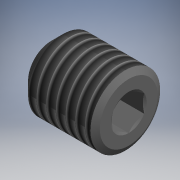
# Autodesk Inventor part: DIN-913 - M18x20
Saved by Autodesk Inventor 2017.3 (Build 213256000, 256)
## iProperties
Part Number: DIN-913 - M18x20
Material: Generic
Catalog Web Link: www.cadenas.de
Description: DIN-913-Gewindestift
Vendor: FESTO
Document SubType Name: Modeling
Designer: partserver
Manufacturer: FESTO
Mass: 4.27109 g
Surface Area: 17.6345 cm^2
Volume: 4.27109 cm^3
Density: 1 g/cm^3
Appearance: PSOLRGB-128-128-128
Category: PARTsolutions
Company: FESTO
Title: DIN-913 - M18x20
Author: Cadenas PARTsolutions
Comments: Gewindestift
PSOL_IDENT_0: {$CADENAS_DATA\23d-libs\festo\zyl_zubeh\din_913\din_913.prj},177 {VTYP=3D},{NB=DIN-913 - M18x20},{LI
PSOL_IDENT_1: NA=DIN-913 - M18x20},{NN=DIN-913},{DATE=22.07.2016 11:33:17},{GEOMDATE=22.07.2016 11:33:13},{VERSION=
PSOL_IDENT_2: v3},{LINEID=1120},{WBVAR=},{WBNUMERIC=}  {NB=DIN-913 - M18x20},{LINA=DIN-913 - M18x20},{KT=X},{IDNR=
PSOL_IDENT_3: },{NENN=M18x20},{D=18.000},{D3=14.933},{P=2.500},{L=20.000},{DP=12.000},{S=8.000},{T=10.000}
NB: DIN-913 - M18x20
NN: DIN-913
NT: Gewindestift
NBSYN: DIN-913 - $NENN.
LINA: DIN-913 - M18x20
CATALOG: Festo
ROWDESC: M18x20
D: 18
D3: 14.933
P: 2.5
L: 20
DP: 12
S: 8
T: 10
SUPPLIER: FESTO
ARTICLENO: DIN-913 - M18x20
BOMINFO: DIN-913 - M18x20
CREATOR: CADENAS GmbH
Autodesk Inventor part; units mm, degrees
sketch "Sketch_1" plane through (0, 0, 0) normal (0, 0, 1) x (1, 0, 0)
  line L0 (2.6667, 0) -> (20, 0)
  line L1 (20, 0) -> (20, -6)
  line L2 (20, -6) -> (17, -9)
  line L3 (17, -9) -> (0.8854, -9)
  line L4 (0.8854, -9) -> (0, -7.4665)
  line L5 (0, -7.4665) -> (0, -4.6188)
  line L6 (0, -4.6188) -> (2.6667, 0)
  line L7 (2.6667, 0) -> (20, 0)
  constraints: 16 end point
revolve "Revolution1" add sketch "Sketch_1" angle 360 about axis through (2.6667, 0, 0) along (1, 0, 0)
thread "Thread1" size "M18x2.5" class "6g" standard "ISO Metric profile" full length
sketch "Sketch_2" plane through (0, 0, 0) normal (1, 0, 0) x (0, 1, 0)
  line L0 (0, 4.6188) -> (-4, 2.3094)
  line L1 (-4, 2.3094) -> (-4, -2.3094)
  line L2 (-4, -2.3094) -> (0, -4.6188)
  line L3 (0, -4.6188) -> (4, -2.3094)
  line L4 (4, -2.3094) -> (4, 2.3094)
  line L5 (4, 2.3094) -> (0, 4.6188)
  constraints: 12 end point
extrude "Extrusion1" cut sketch "Sketch_2" along normal blind 10
ref_plane "IP1_XY" through (0, 0, 0) normal (1, 0, 0) x (0, 0, -1)
ref_plane "IP1_YZ" through (0, 0, 0) normal (0, 0, -1) x (0, 1, 0)
ref_plane "IP1_ZX" through (0, 0, 0) normal (0, 1, 0) x (1, 0, 0)
ref_plane "IP2_XY" through (20, 0, 0) normal (1, 0, 0) x (0, 0, -1)
ref_plane "IP2_YZ" through (20, 0, 0) normal (0, 0, -1) x (0, 1, 0)
ref_plane "IP2_ZX" through (20, 0, 0) normal (0, 1, 0) x (1, 0, 0)
body "Solid1"
